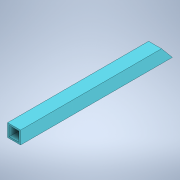
# Autodesk Inventor part: Aluminum1x1MiddleBack
Saved by Autodesk Inventor 2020.2 (Build 242310000, 310)
## iProperties
Created: 2020-01-26
Part Number: Aluminum1x1MiddleBack
Material: Aluminum 6061
Document SubType Name: Modeling
Designer: robst
Density: 2.7 g/cm^3
Appearance: Cadet Blue
Author: robst
Autodesk Inventor part; units mm, degrees
ref_plane "YZ Plane" through (0, 0, 0) normal (1, 0, 0) x (0, 1, 0)
ref_plane "XZ Plane" through (0, 0, 0) normal (0, 1, 0) x (-1, 0, 0)
ref_plane "XY Plane" through (0, 0, 0) normal (0, 0, 1) x (1, 0, 0)
sketch "Sketch1" plane through (0, 0, 0) normal (0, 0, 1) x (1, 0, 0)
  line L0 (-12.7, -12.7) -> (12.7, -12.7)
  line L1 (12.7, -12.7) -> (12.7, 12.7)
  line L2 (12.7, 12.7) -> (-12.7, 12.7)
  line L3 (-12.7, 12.7) -> (-12.7, -12.7)
  line L4 (-12.7, -12.7) -> (12.7, 12.7) construction
  line L5 (12.7, -12.7) -> (-12.7, 12.7) construction
  line L6 (-9.525, -9.525) -> (9.525, -9.525)
  line L7 (9.525, -9.525) -> (9.525, 9.525)
  line L8 (9.525, 9.525) -> (-9.525, 9.525)
  line L9 (-9.525, 9.525) -> (-9.525, -9.525)
  line L10 (-9.525, -9.525) -> (9.525, 9.525) construction
  line L11 (9.525, -9.525) -> (-9.525, 9.525) construction
  point P0 (0, 0)
  dimension "d0" = 25.4
  dimension "d1" = 25.4
  dimension "d2" = 3.175
  constraints: 24 end point, 5 parallel, 4 midpoint, 3 perpendicular, 1 horizontal
  measures "d0" distance of L0.start L0.end
  measures "d1" distance of L1.end L0.end
  measures "d2" distance between parallel lines of L0 L6
extrude "Extrusion1" add sketch "Sketch1" along normal mid plane 298.45
sketch "Sketch4" plane through (12.7, -12.7, 149.225) normal (1, 0, 0) x (0, 0, -1)
  line L0 (298.45, 0) -> (298.45, 25.4) projected
  line L1 (298.45, 0) -> (277.1369, 25.4)
  line L2 (298.45, 25.4) -> (0, 25.4) projected
  line L3 (277.1369, 25.4) -> (298.45, 25.4)
  line L4 (298.45, 22.225) -> (0, 22.225) projected
  line L5 (298.45, 25.4) -> (298.45, 0)
  point P0 (149.225, 12.7)
  dimension "d9" = 40
  constraints: 6 end point, 1 parallel, 1 perpendicular, 1 point on line
  measures "d9" angle of L1 L0
extrude "Extrusion3" cut sketch "Sketch4" against normal through all
body "Solid1"
